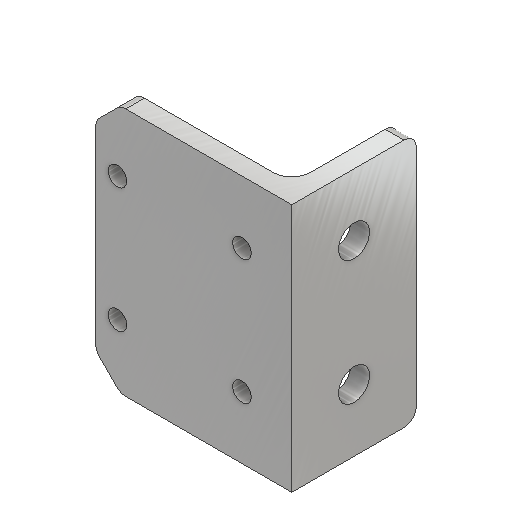
# Autodesk Inventor part: CNCM_ALU_X_Y_AXis_Mounting_Bracket
Saved by Autodesk Inventor 2026.1 (Build 301233000, 233)
## iProperties
Created: 2016-03-27
Part Number: CNCM_ALU_X_Y_AXis_Mounting_Bracket
Material: Ogólny
Document SubType Name: Modeling
Designer: Andrzej
Density: 1 g/cm^3
Appearance: Obrobione - aluminium
Mass: 5.64009 g
Surface Area: 43.803 cm^2
Volume: 5.64009 cm^3
Author: Andrzej
Autodesk Inventor part; units mm, degrees
ref_plane "YZ Plane" through (0, 0, 0) normal (1, 0, 0) x (0, 1, 0)
ref_plane "XZ Plane" through (0, 0, 0) normal (0, 1, 0) x (-1, 0, 0)
ref_plane "XY Plane" through (0, 0, 0) normal (0, 0, 1) x (1, 0, 0)
sketch "Szkic1" plane through (0, 0, 0) normal (0, 0, 1) x (1, 0, 0)
  line L0 (-15.1556, -3.6171) -> (-15.1556, -6.6171)
  line L1 (-15.1556, -6.6171) -> (16.3444, -6.6171)
  line L2 (16.3444, -6.6171) -> (16.3444, 13.3829)
  line L3 (16.3444, 13.3829) -> (13.3444, 13.3829)
  line L4 (13.3444, 13.3829) -> (13.3444, -3.6171)
  line L5 (13.3444, -3.6171) -> (-15.1556, -3.6171)
  point P0 (0, 0)
  dimension "d0" = 3
  dimension "d1" = 31.5
  dimension "d2" = 20
  dimension "d3" = 3
  constraints: 12 end point, 5 perpendicular, 1 vertical
  measures "d0" distance of L0.start L0.end
  measures "d1" distance of L0.end L1.end
  measures "d2" distance of L1.end L2.end
  measures "d3" distance of L2.end L3.end
extrude "Wyciągnięcie proste1" add sketch "Szkic1" along normal blind 40
fillet "Zaokrąglenie1" radius 3 1 edges at (13.3444, -3.6171, 20)
fillet "Zaokrąglenie3" radius 2 2 edges at (14.8444, 13.3829, 40) (14.8444, 13.3829, 0)
sketch "Szkic4" plane through (-15.1556, -6.6171, 0) normal (0, -1, 0) x (1, 0, 0)
  line L0 (0, 0) -> (31.5, 0) projected
  line L1 (31.5, 0) -> (31.5, 40) projected
  line L2 (0, 40) -> (31.5, 40) projected
  line L3 (0, 0) -> (0, 40) projected
  line L4 (31.5, 36.2) -> (-0.3213, 36.2)
  line L5 (31.5, 2) -> (31.5, 38) projected
  line L6 (31.5, 3.8) -> (0, 3.8)
  line L7 (0, 0) -> (0, 40) projected
  line L8 (27, 36.2) -> (27, 3.8)
  point P0 (15.1556, 0)
  point P1 (23.5, 30)
  point P2 (3.5, 30)
  point P3 (23.5, 10)
  point P4 (3.5, 10)
  dimension "d47" = 32.4
  dimension "d48" = 3.8
  dimension "d50" = 3.5
  dimension "d51" = 3.5
  dimension "d53" = 6.2
  dimension "d54" = 6.2
  dimension "d55" = 6.2
  dimension "d56" = 6.2
  dimension "d68" = 4.5
  dimension "d69" = 3.5
  dimension "d70" = 3.5
  dimension "d78" = 27
  constraints: 6 end point, 5 point on line, 3 perpendicular
  measures "d47" distance between parallel lines of L6 L4
  measures "d48" distance between parallel lines of L0 L6
  measures "d50" distance from line of L3 point (3.5, 30)
  measures "d51" distance from line of L3 point (3.5, 10)
  measures "d53" distance from line of L4 point (23.5, 30)
  measures "d54" distance from line of L4 point (3.5, 30)
  measures "d55" distance from line of L6 point (3.5, 10)
  measures "d56" distance from line of L6 point (23.5, 10)
  measures "d68" distance between parallel lines of L1 L8
  measures "d69" distance from line of L8 point (23.5, 30)
  measures "d70" distance from line of L8 point (23.5, 10)
  measures "d78" distance between parallel lines of L3 L8
sketch "Szkic5" plane through (16.3444, -6.6171, 40) normal (1, 0, 0) x (0, 0, -1)
  arc A0 (40, 18) -> (38, 20) centre (38, 18) ccw projected
  line L0 (38, 20) -> (2, 20) projected
  arc A1 (2, 20) -> (0, 18) centre (2, 18) ccw projected
  line L1 (0, 0) -> (0, 18) projected
  line L2 (40, 0) -> (0, 0) projected
  line L3 (40, 0) -> (40, 18) projected
  point P0 (40, 6.6171)
  point P1 (10, 10)
  point P2 (30, 10)
  dimension "d57" = 10
  dimension "d58" = 10
  dimension "d59" = 10
  dimension "d60" = 10
  measures "d57" distance from line of L0 point (10, 10)
  measures "d58" distance from line of L1 point (10, 10)
  measures "d59" distance from line of L0 point (30, 10)
  measures "d60" distance from line of L3 point (30, 10)
hole "Otwór3" at (16.3444, 3.3829, 30) at (16.3444, 3.3829, 10) direction (-1, 0, 0) diameter 5 end through all
hole "Otwór4" at (8.3444, -6.6171, 30) at (-11.6556, -6.6171, 30) at (8.3444, -6.6171, 10) at (-11.6556, -6.6171, 10) direction (0, 1, 0) diameter 3 end through all
sketch "Szkic6" plane through (-15.1556, -3.6171, 40) normal (0, 1, 0) x (1, 0, 0)
  circle A0 centre (23.5, 10) radius 1.5 projected
  circle A1 centre (23.5, 30) radius 1.5 projected
  circle A2 centre (23.5, 10) radius 1.5 projected
  circle A3 centre (23.5, 10) radius 3.1
  circle A4 centre (23.5, 30) radius 3.1
  point P0 (15.1556, 40)
  dimension "d79" = 6.2
  dimension "d80" = 6.2
  constraints: 2 centre point, 2 coincident
  measures "d79" diameter of A3
  measures "d80" diameter of A4
extrude "Wyciągnięcie proste3" cut sketch "Szkic6" along normal blind 10
chamfer "Faza3" distance 4 angle 45 2 edges at (-15.1556, -5.1171, 40) (-15.1556, -5.1171, 0)
fillet "Zaokrąglenie4" radius 2 4 edges at (-15.1556, -5.1171, 36) (-11.1556, -5.1171, 40) (-15.1556, -5.1171, 4) (-11.1556, -5.1171, 0)
equation "\"d50\" = d69"
equation "\"d51\" = d69"
equation "\"d54\" = d53"
equation "\"d55\" = d53"
equation "\"d56\" = d53"
equation "\"d70\" = d69"
equation "\"d58\" = d57"
equation "\"d59\" = d57"
equation "\"d60\" = d59"
